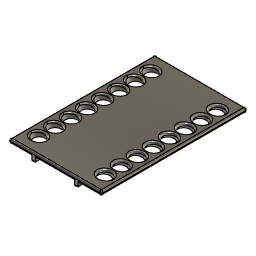
PCRtubeMagnetHolder2 (Autodesk Fusion 360 design; units mm, degrees)
Autodesk Fusion 360 part; units mm, degrees
note: some values were not read from the file. Set by a fixed rule: which sketch regions a step uses; which face or edge a step refers to.
sketch "Sketch1" plane through (0, 0, 0) normal (0, 0, 1) x (1, 0, 0)
  line L0 (0, 0) -> (11, 0)
  line L1 (11, 0) -> (11, 82)
  line L2 (11, 82) -> (0, 82)
  line L3 (0, 82) -> (0, 0)
  line L4 (11, 0) -> (26, 0)
  line L5 (26, 0) -> (26, 82)
  line L6 (26, 82) -> (11, 82)
  line L7 (11, 82) -> (11, 0)
  line L8 (11, 82) -> (13, 82)
  line L9 (13, 82) -> (13, 0)
  line L10 (13, 0) -> (11, 0)
  line L11 (11, 0) -> (11, 82)
  dimension "d1" = 11
  dimension "d2" = 82
  dimension "d3" = 15
  dimension "d4" = 82
  dimension "d7" = 2
  dimension "d8" = 82
  constraint horizontal L0
  constraint vertical L1
  constraint horizontal L2
  constraint vertical L3
  constraint coincident L0.start L3.end
  constraint horizontal L4
  constraint vertical L5
  constraint horizontal L6
  constraint vertical L7
  constraint horizontal L8
  constraint vertical L9
  constraint horizontal L10
  constraint vertical L11
  measures "d1" distance of L0.start L0.end
  measures "d2" distance of L0.start L2.end
  measures "d3" distance of L0.end L4.end
  measures "d4" distance of L0.end L1.end
  measures "d7" distance of L1.end L8.end
  measures "d8" distance of L1.end L0.end
extrude "Extrude1" add sketch "Sketch1" along normal blind 2.5
sketch "Sketch2" plane through (0, 0, 0) normal (0, -1, 0) x (1, 0, 0)
  line L0 (26, 2.5) -> (0, 2.5)
  line L1 (0, 2.5) -> (0, 0)
  line L2 (0, 0) -> (26, 0)
  line L3 (26, 0) -> (26, 2.5)
  line L4 (26, 0) -> (26, 2.5)
  line L5 (26, 2.5) -> (13.9338, 8.1265)
  line L6 (26, 2.5) -> (19.5247, 1.9335)
  line L7 (19.5247, 1.9335) -> (19.1977, 5.672)
  dimension "d11" = 115
  constraint coincident L2.end L3.start
  constraint coincident L0.start L3.end
  constraint coincident L5 L7.end
  constraint perpendicular L6 L7
  measures "d11" angle of L4 L5
ref_plane "WorkPlane1" through (19.9669, 0, 5.3133) normal (0.422618, 0, 0.906308) x (-0.906308, 0, 0.422618)
sketch "Sketch3" plane through (19.9669, 0, 5.3133) normal (0.422618, 0, 0.906308) x (-0.906308, 0, 0.422618)
  line L0 (-0.5, 0) -> (-0.5, -82)
  line L1 (-0.5, 0) -> (-0.5, -9.5) construction
  circle A0 centre (-0.5, -9.5) radius 3.25
  circle A1 centre (-0.5, -18.5) radius 3.25
  circle A2 centre (-0.5, -36.5) radius 3.25
  circle A3 centre (-0.5, -27.5) radius 3.25
  circle A4 centre (-0.5, -72.5) radius 3.25
  circle A5 centre (-0.5, -63.5) radius 3.25
  circle A6 centre (-0.5, -54.5) radius 3.25
  circle A7 centre (-0.5, -45.5) radius 3.25
  dimension "d13" = 82
  dimension "d14" = 9.5
  dimension "d15" = 6.5
  dimension "d16" = 6.5
  dimension "d17" = 9
  dimension "d18" = 6.5
  dimension "d19" = 6.5
  dimension "d20" = 9
  dimension "d21" = 9
  dimension "d22" = 6.5
  dimension "d23" = 6.5
  dimension "d24" = 9
  dimension "d25" = 6.5
  dimension "d26" = 6.5
  dimension "d27" = 9
  dimension "d28" = 9
  dimension "d29" = 9
  dimension "d30" = 9.5
  constraint vertical L0
  constraint parallel L0 L1
  constraint coincident L1.end A0.centre
  measures "d13" distance of L0.start L0.end
  measures "d14" distance of L0.start L1.end
  measures "d15" diameter of A0
  measures "d16" diameter of A1
  measures "d17" distance of L1.end A1.centre
  measures "d18" diameter of A3
  measures "d19" diameter of A2
  measures "d20" distance of A3.centre A2.centre
  measures "d21" distance of A1.centre A3.centre
  measures "d22" diameter of A7
  measures "d23" diameter of A6
  measures "d24" distance of A7.centre A6.centre
  measures "d25" diameter of A5
  measures "d26" diameter of A4
  measures "d27" distance of A5.centre A4.centre
  measures "d28" distance of A5.centre A6.centre
  measures "d29" distance of A2.centre A7.centre
  measures "d30" distance of L0.end A4.centre
extrude "Extrude3" cut sketch "Sketch3" against normal blind 15
extrude "Extrude4" add sketch "Sketch1" against normal blind 2.5 contours L1 L4 L6 L7 L8 L9 L10 L11
mirror "Mirror1" about plane through (0, 82, 0) normal (-1, 0, 0) of bodies 1 merged
fillet "Fillet1" radius 1 1 faces at (-5.8102, 79.7745, 2.5)
fillet "Fillet1" radius 1 2 faces at (11.6667, 27.3333, -2.5) (-11.6667, 27.3333, -2.5)
fillet "Fillet1" radius 1 12 edges at (-26, 41, 0) (-19.5, 0, 0) (0, 0, 0) (19.5, 0, 0) (26, 41, 0) (-26, 0, 1.25) (26, 0, 1.25) (19.5, 82, 0) (0, 82, 0) (-19.5, 82, 0) (-26, 82, 1.25) (26, 82, 1.25)
